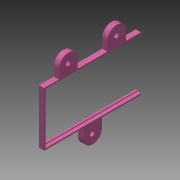
# Autodesk Inventor part: Part11
Saved by Autodesk Inventor 2015 (Build 190159000, 159)
## iProperties
Created: 2015-07-08
Part Number: Part11
Material: ABS Plastic
Document SubType Name: Modeling
Designer: eefred
Density: 1.06 g/cm^3
Appearance: Pink
Author: eefred
Autodesk Inventor part; units mm, degrees
ref_plane "YZ Plane" through (0, 0, 0) normal (1, 0, 0) x (0, 1, 0)
ref_plane "XZ Plane" through (0, 0, 0) normal (0, 1, 0) x (-1, 0, 0)
ref_plane "XY Plane" through (0, 0, 0) normal (0, 0, 1) x (1, 0, 0)
sketch "Sketch1" plane through (0, 0, 0) normal (1, 0, 0) x (0, 1, 0)
  line L0 (0, 29) -> (103.5, 29)
  line L1 (103.5, -29) -> (0, -29)
  line L2 (0, -29) -> (0, 29)
  line L3 (103.5, 29) -> (103.5, 26.5)
  line L4 (103.5, 26.5) -> (3, 26.5)
  line L5 (3, 26.5) -> (3, -26.5)
  line L6 (3, -26.5) -> (103.5, -26.5)
  line L7 (103.5, -26.5) -> (103.5, -29)
  point P0 (0, 0)
  point P1 (0, 0)
  dimension "d0" = 103.5
  dimension "d1" = 58
  dimension "d2" = 2.5
  dimension "d3" = 2.5
  dimension "d4" = 3
  constraints: 16 end point, 4 perpendicular, 1 coincident, 1 horizontal, 1 midpoint, 1 parallel, 1 point on line, 1 vertical, 1 vertical alignment
  measures "d0" distance of L1.start L1.end
  measures "d1" distance of L0.end L1.start
  measures "d2" distance of L0.end L3.end
  measures "d3" distance of L6.end L1.start
  measures "d4" distance between parallel lines of L2 L5
extrude "Extrusion1" add sketch "Sketch1" along normal blind 5.5
sketch "Sketch2" plane through (5.5, 0, 0) normal (1, 0, 0) x (0, 0, -1)
  circle A0 centre (39, 51.75) radius 2.5
  circle A1 centre (-39, 77.63) radius 2.5
  circle A2 centre (-39, 25.88) radius 2.5
  arc A3 (39, 41.75) -> (39, 61.75) centre (39, 51.75) ccw
  arc A4 (-39, 87.63) -> (-39, 67.63) centre (-39, 77.63) ccw
  arc A5 (-39, 35.88) -> (-39, 15.88) centre (-39, 25.88) ccw
  line L0 (-39, 87.63) -> (-29, 87.63)
  line L1 (-29, 87.63) -> (-29, 67.63)
  line L2 (-29, 67.63) -> (-39, 67.63)
  line L3 (-39, 35.88) -> (-29, 35.88)
  line L4 (-29, 35.88) -> (-29, 15.88)
  line L5 (-29, 15.88) -> (-39, 15.88)
  line L6 (39, 41.75) -> (29, 41.75)
  line L7 (29, 41.75) -> (29, 61.75)
  line L8 (29, 61.75) -> (39, 61.75)
  point P0 (0, 0)
  point P1 (-29, 0)
  point P2 (29, 0)
  dimension "d9" = 5
  dimension "d10" = 10
  dimension "d11" = 10
  dimension "d12" = 41.75
  dimension "d13" = 15.88
  dimension "d14" = 51.75
  constraints: 18 end point, 7 point on circle, 6 centre point, 6 perpendicular, 6 tangent, 4 equal radius, 3 coincident, 3 horizontal, 3 vertical alignment, 2 parallel
  measures "d9" diameter of A0
  measures "d10" radius of A3
  measures "d11" distance of L6.start L6.end
  measures "d12" distance from line of point (0, 0) L6
  measures "d13" distance from line of point (0, 0) L5
  measures "d14" distance between parallel lines of L5 L2
extrude "Extrusion2" add sketch "Sketch2" against normal blind 5.5
sketch "Sketch3" plane through (5.5, 0, 0) normal (1, 0, 0) x (0, 0, -1)
  line L0 (-27.5, 103.5) -> (27.5, 103.5)
  line L1 (27.5, 103.5) -> (27.5, 1.5)
  line L2 (27.5, 1.5) -> (-27.5, 1.5)
  line L3 (-27.5, 1.5) -> (-27.5, 103.5)
  line L4 (-26.5, 3) -> (-26.5, 103.5) projected
  line L5 (26.5, 103.5) -> (26.5, 3) projected
  line L6 (26.5, 3) -> (-26.5, 3) projected
  point P0 (0, 0)
  point P1 (-29, 103.5)
  dimension "d17" = 1
  dimension "d18" = 1
  dimension "d19" = 1.5
  constraints: 8 end point, 2 parallel, 1 horizontal, 1 horizontal alignment, 1 perpendicular
  measures "d17" distance between parallel lines of L4 L3
  measures "d18" distance between parallel lines of L5 L1
  measures "d19" distance between parallel lines of L6 L2
extrude "Extrusion3" cut sketch "Sketch3" against normal blind 3.5
equation "\"d3\" = d2"
equation "\"d18\" = d17"
body "Solid1"
